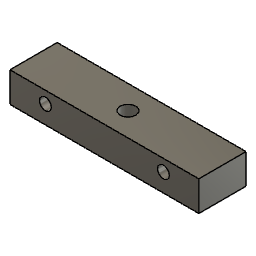
CableClampBracket v8 (Autodesk Fusion 360 archive; units mm, degrees)
design "CableClampBracket" references "tormach 770mx"
Autodesk Fusion 360 part; units mm, degrees
sketch "Sketch1" plane through (0, 0, 0) normal (0, 1, 0) x (1, 0, 0)
  line L0 (0, 0) -> (40, 0)
  line L1 (40, 0) -> (40, -10)
  line L2 (40, -10) -> (0, -10)
  line L3 (0, -10) -> (0, 0)
  dimension "d1" = 40
  dimension "d2" = 10
  constraint horizontal L0
  constraint vertical L1
  constraint horizontal L2
  constraint vertical L3
  constraint coincident L0.start L3.end
  measures "d1" distance of L0.start L0.end
  measures "d2" distance of L0.start L2.end
extrude "Extrude1" add sketch "Sketch1" along normal blind 6.35
sketch "Sketch2" plane through (0, 6.35, 0) normal (0, 1, 0) x (-1, 0, 0)
  line L0 (0, 10) -> (-40, 10)
  line L1 (-40, 10) -> (-40, 0)
  line L2 (-40, 0) -> (0, 0)
  line L3 (0, 0) -> (0, 10)
  line L4 (0, 5) -> (-40, 5) construction
  point P0 (-20, 5)
  constraint midpoint L3 L4.start
  constraint midpoint L1 L4.end
  constraint midpoint L4 P0
hole "Hole1" at (20, 6.35, 5) direction (0, -1, 0) diameter 3.3 end through all
sketch "Sketch3" plane through (0, 0, 10) normal (0, 0, 1) x (1, 0, 0)
  line L0 (0, 0) -> (40, 0)
  line L1 (40, 0) -> (40, 6.35)
  line L2 (40, 6.35) -> (0, 6.35)
  line L3 (0, 6.35) -> (0, 0)
  line L4 (0, 3.85) -> (39.5878, 3.85) construction
  point P0 (7.5, 3.85)
  point P1 (32.5, 3.85)
  dimension "d10" = 7.5
  dimension "d11" = 25
  dimension "d18" = 2.5
  constraint coincident L4 P0
  constraint coincident L4 P1
  measures "d10" distance of L3 P0
  measures "d11" distance of P0 P1
  measures "d18" distance of L2 L4
hole "Hole4" at (7.5, 3.85, 10) direction (0, 0, -1) diameter 2.5 end through all
hole "Hole5" at (32.5, 3.85, 10) direction (0, 0, -1) diameter 2.5 end through all
hole "Hole2" [suppressed]
hole "Hole3" [suppressed]
